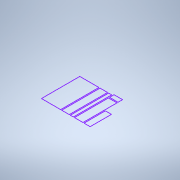
# Autodesk Inventor part: soiya
Saved by Autodesk Inventor 2022 (Build 260153000, 153)
## iProperties
Created: 2023-01-17
Part Number: soiya
Material: 一般
Document SubType Name: Modeling
Designer: tdn82
Density: 1 g/cm^3
Appearance: 既定
Author: tdn82
Autodesk Inventor part; units mm, degrees
ref_plane "YZ Plane" through (0, 0, 0) normal (1, 0, 0) x (0, 1, 0)
ref_plane "XZ Plane" through (0, 0, 0) normal (0, 1, 0) x (-1, 0, 0)
ref_plane "XY Plane" through (0, 0, 0) normal (0, 0, 1) x (1, 0, 0)
sketch "スケッチ1" plane through (0, 0, 0) normal (0, 1, 0) x (-1, 0, 0)
  line L0 (0, 0) -> (-500, 0)
  line L1 (-500, 0) -> (-500, -500)
  line L2 (-500, -500) -> (0, -500)
  line L3 (0, -500) -> (0, 0)
  dimension "d0" = 500
  dimension "d1" = 500
  constraints: 8 end point, 2 parallel, 1 horizontal, 1 perpendicular
  measures "d0" distance of L2.end L0.start
  measures "d1" distance of L0.start L0.end
extrude "押し出し1" add sketch "スケッチ1" along normal blind 2
sketch "スケッチ2" plane through (0, 2, 0) normal (0, 1, 0) x (1, 0, 0)
  line L0 (0, 0) -> (180, 0)
  line L1 (180, 0) -> (180, 360)
  line L2 (180, 360) -> (0, 360)
  line L3 (0, 360) -> (0, 0)
  line L4 (190, 0) -> (261, 0)
  line L5 (261, 0) -> (261, 360)
  line L6 (261, 360) -> (190, 360)
  line L7 (190, 360) -> (190, 0)
  line L8 (271, 0) -> (300, 0)
  line L9 (300, 0) -> (300, 360)
  line L10 (300, 360) -> (271, 360)
  line L11 (271, 360) -> (271, 0)
  line L12 (310, 0) -> (390, 0)
  line L13 (390, 0) -> (390, 319.5)
  line L14 (390, 319.5) -> (310, 319.5)
  line L15 (310, 319.5) -> (310, 0)
  line L16 (310, 329.5) -> (390, 329.5)
  line L17 (390, 329.5) -> (390, 372)
  line L18 (390, 372) -> (310, 372)
  line L19 (310, 372) -> (310, 329.5)
  line L20 (400, 0) -> (457.5, 0)
  line L21 (457.5, 0) -> (457.5, 200)
  line L22 (457.5, 200) -> (400, 200)
  line L23 (400, 200) -> (400, 0)
  dimension "d4" = 360
  dimension "d5" = 180
  dimension "d6" = 71
  dimension "d7" = 10
  dimension "d8" = 29
  dimension "d9" = 10
  dimension "d10" = 319.5
  dimension "d11" = 80
  dimension "d12" = 10
  dimension "d13" = 42.5
  dimension "d14" = 10
  dimension "d16" = 57.5
  dimension "d17" = 10
  constraints: 48 end point, 12 parallel, 6 horizontal, 6 perpendicular
  measures "d4" distance of L0.end L1.end
  measures "d5" distance of L1.end L2.end
  measures "d6" distance of L5.end L6.end
  measures "d7" distance between parallel lines of L7 L1
  measures "d8" distance between parallel lines of L9 L11
  measures "d9" distance between parallel lines of L11 L5
  measures "d10" distance of L14.end L12.start
  measures "d11" distance of L13.end L14.end
  measures "d12" distance between parallel lines of L15 L9
  measures "d13" distance of L18.end L16.start
  measures "d14" distance between parallel lines of L14 L16
  measures "d16" distance of L21.end L22.end
  measures "d17" distance between parallel lines of L23 L13
